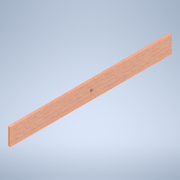
# Autodesk Inventor part: Querstrebe_camera
Saved by Autodesk Inventor 2021 (Build 250183000, 183)
## iProperties
Created: 2022-06-26
Part Number: Querstrebe_camera
Material: Holz (Eiche)
Document SubType Name: Modeling
Designer: adria
Density: 0.76 g/cm^3
Appearance: Weißeiche - natur - mittlerer Glanz
Mass: 57.6526 g
Surface Area: 346.377 cm^2
Volume: 75.8586 cm^3
Author: adria
Autodesk Inventor part; units mm, degrees
ref_plane "YZ Plane" through (0, 0, 0) normal (1, 0, 0) x (0, 1, 0)
ref_plane "XZ Plane" through (0, 0, 0) normal (0, 1, 0) x (-1, 0, 0)
ref_plane "XY Plane" through (0, 0, 0) normal (0, 0, 1) x (1, 0, 0)
sketch "Skizze1" plane through (0, 0, 0) normal (0, 0, 1) x (1, 0, 0)
  line L0 (-2.5, -20) -> (2.5, -20)
  line L1 (2.5, -20) -> (2.5, 20)
  line L2 (2.5, 20) -> (-2.5, 20)
  line L3 (-2.5, 20) -> (-2.5, -20)
  line L4 (-2.5, -20) -> (2.5, 20) construction
  line L5 (2.5, -20) -> (-2.5, 20) construction
  point P0 (0, 0)
  dimension "d0" = 5
  dimension "d1" = 40
  constraints: 12 end point, 2 midpoint, 2 parallel, 1 horizontal, 1 perpendicular
  measures "d0" distance of L2.end L1.end
  measures "d1" distance of L1.end L0.end
extrude "Extrusion1" add sketch "Skizze1" along normal blind 380
sketch "Skizze2" plane through (2.5, -20, 0) normal (1, 0, 0) x (0, 0, -1)
  line L0 (0, 0) -> (0, 40) projected
  line L1 (0, 40) -> (-380, 40) projected
  line L2 (-380, 0) -> (-380, 40) projected
  line L3 (0, 0) -> (-380, 0) projected
  point P0 (0, 20)
  point P1 (-190, 20)
  point P2 (0, 20)
  dimension "d4" = 380
  dimension "d5" = 190
  constraints: 1 horizontal alignment, 1 midpoint
  measures "d4" distance between parallel lines of L0 L2
  measures "d5" distance from line of L2 point (-190, 20)
hole "Bohrung1" at (2.5, 0, 190) direction (-1, 0, 0) diameter 6 end through all
equation "\"d5\" = 0.5 * d4"
